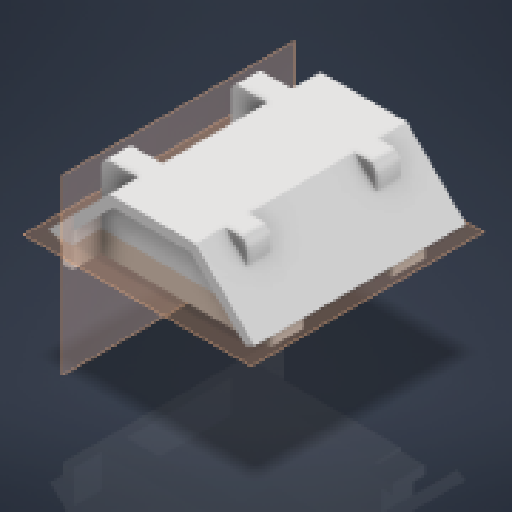
# Autodesk Inventor part: КрышкаЕСК
Saved by Autodesk Inventor 2026 (Build 300175000, 175)
## iProperties
Created: 2025-08-21
Part Number: КрышкаЕСК
Material: Типовые
Document SubType Name: Modeling
Designer: seraf
Density: 1 g/cm^3
Appearance: По умолчанию
Author: seraf
Autodesk Inventor part; units mm, degrees
ref_plane "XY Plane" through (0, 0, 0) normal (0, 0, 1) x (1, 0, 0)
sketch "Эскиз1" plane through (0, 0, 0) normal (0, 0, 1) x (1, 0, 0)
  line L0 (21.7279, 9) -> (24, 10) projected
  line L1 (10, 24) -> (24, 10) projected
  line L2 (-10, 24) -> (10, 24) projected
  line L3 (-24, 10) -> (-10, 24) projected
  line L4 (-24, 10) -> (-21.7279, 9) projected
  line L5 (-9, 21.7279) -> (-21.7279, 9) projected
  line L6 (9, 21.7279) -> (-9, 21.7279) projected
  line L7 (21.7279, 9) -> (9, 21.7279) projected
  point P0 (0, 0)
ref_plane "РабПлоскость1" through (-24, 9, 50) normal (0, 0, -1) x (0, 1, 0)
extrude "Выдавливание1" add sketch "Эскиз1" along normal up to surface (50 mm away)
sketch "Эскиз2" plane through (0, 0, 0) normal (0, 0, -1) x (-1, 0, 0)
  line L0 (-21.7279, 9) -> (-24, 10) projected
  line L1 (-10, 24) -> (-24, 10) projected
  line L2 (10, 24) -> (-10, 24) projected
  line L3 (24, 10) -> (10, 24) projected
  line L4 (24, 10) -> (21.7279, 9) projected
  line L5 (9, 21.7279) -> (21.7279, 9) projected
  line L6 (-9, 21.7279) -> (9, 21.7279) projected
  line L7 (-21.7279, 9) -> (-9, 21.7279) projected
  point P0 (0, 0)
extrude "Выдавливание2" cut sketch "Эскиз2" against normal blind 0.5
sketch "Эскиз4" plane through (-10, 24, 50) normal (0, 0, 1) x (1, 0, 0)
  line L0 (19, -2.2721) -> (31.7279, -15) projected
  line L1 (31.7279, -15) -> (34, -14) projected
  line L2 (34, -14) -> (20, 0) projected
  line L3 (20, 0) -> (0, 0) projected
  line L4 (0, 0) -> (-14, -14) projected
  line L5 (-14, -14) -> (-11.7279, -15) projected
  line L6 (-11.7279, -15) -> (1, -2.2721) projected
  line L7 (1, -2.2721) -> (19, -2.2721) projected
  point P0 (10, -24)
extrude "Выдавливание4" cut sketch "Эскиз4" against normal blind 0.5
ref_plane "РабПлоскость3" through (-18.5, 0, 0) normal (1, 0, 0) x (0, 1, 0)
sketch "Эскиз6" plane through (-18.5, 0, 0) normal (1, 0, 0) x (0, 1, 0)
  circle A0 centre (7.1085, 40) radius 1.5 projected
  circle A1 centre (7.1085, 10) radius 1.5 projected
  line L0 (-9, 55) -> (9, 55) construction
  line L1 (-9, 55) -> (-9, -15) construction
  line L2 (9, -15) -> (-9, -15) construction
  line L3 (9, 0) -> (9, -15) construction
  line L4 (9, 50) -> (9, 0) construction
  line L5 (9, 55) -> (9, 50) construction
  line L6 (9, 0.5) -> (9, 49.5) projected
  line L7 (9, 49.5) -> (4.5, 49.5)
  line L8 (4.5, 49.5) -> (4.5, 0.5)
  line L9 (4.5, 0.5) -> (9, 0.5)
  line L10 (9, 0.5) -> (9, 49.5)
  point P0 (0, 0)
  dimension "d10" = 4.5
  constraints: 8 end point, 2 parallel, 1 horizontal, 1 perpendicular
  measures "d10" distance of L9.end L8.end
extrude "Выдавливание5" add sketch "Эскиз6" against normal blind 2.5
sketch "Эскиз7" plane through (-18.5, 9, 49.5) normal (0, 1, 0) x (1, 0, 0)
  line L0 (0, 49) -> (0, 0) projected
  line L1 (0, 49) -> (-2.5, 49) projected
  line L2 (-2.5, 0) -> (-2.5, 49) projected
  line L3 (0, 0) -> (-2.5, 0) projected
  point P0 (18.5, 49.5)
extrude "Выдавливание6" add sketch "Эскиз7" along normal up to surface surface through (-21.7279, 9, 0) normal (0.7071068, -0.7071068, 0)
sketch "Эскиз8" plane through (-21.7279, 9, 49.5) normal (0.7071068, -0.7071068, 0) x (-0.7071068, -0.7071068, 0)
  line L0 (-1.0294, 49) -> (-1.0294, 0) projected
  line L1 (-1.0294, 0) -> (0, 0) projected
  line L2 (0, 49) -> (0, 0) projected
  line L3 (0, 49) -> (-1.0294, 49) projected
  point P0 (-9, 49.5)
extrude "Выдавливание7" add sketch "Эскиз8" along normal up to surface surface through (-21, 6.75, 25) normal (1, 0, 0)
sketch "Эскиз9" plane through (-21, 7.1085, 10) normal (1, 0, 0) x (0, 0, -1)
  circle A0 centre (-30, 0) radius 1.5 projected
  circle A1 centre (0, 0) radius 1.5 projected
  point P0 (10, -7.1085)
extrude "Выдавливание8" cut sketch "Эскиз9" against normal blind 10
ref_plane "РабПлоскость4" through (0, 9.5, 0) normal (0, 1, 0) x (-1, 0, 0)
sketch "Эскиз10" plane through (0, 9.5, 0) normal (0, 1, 0) x (-1, 0, 0)
  line L0 (-21.7279, 15.2) -> (-21.7279, 6.8) construction
  line L1 (-21.7279, 43.2) -> (-21.7279, 34.8) construction
  line L2 (-18.7279, 6.8) -> (-18.7279, 15.2) construction
  line L3 (-18.7279, 34.8) -> (-18.7279, 43.2) construction
  line L4 (-18.2279, 7.2) -> (-15.2279, 7.2)
  line L5 (-15.2279, 7.2) -> (-15.2279, 14.8)
  line L6 (-15.2279, 14.8) -> (-18.2279, 14.8)
  line L7 (-18.2279, 14.8) -> (-18.2279, 7.2)
  line L8 (-18.2279, 35.2) -> (-15.2279, 35.2)
  line L9 (-15.2279, 35.2) -> (-15.2279, 42.8)
  line L10 (-15.2279, 42.8) -> (-18.2279, 42.8)
  line L11 (-18.2279, 42.8) -> (-18.2279, 35.2)
  line L12 (-18.7279, 14.8) -> (-18.2279, 14.8) construction
  line L13 (-18.7279, 42.8) -> (-18.2279, 42.8) construction
  line L14 (-24, 55) -> (-24, -15) construction
  point P0 (0, 0)
  dimension "d20" = 0.5
  dimension "d21" = 3
  dimension "d26" = 7.6
  dimension "d27" = 0.4
  dimension "d28" = 0.4
  dimension "d29" = 7.6
  constraints: 20 end point, 6 parallel, 4 horizontal, 2 perpendicular, 2 point on line
  measures "d20" distance of L12.start L6.end
  measures "d21" distance of L5.end L6.end
  measures "d26" distance of L4.end L5.end
  measures "d27" distance of L2.end L12.start
  measures "d28" distance of L3.end L13.start
  measures "d29" distance of L8.end L9.end
extrude "Выдавливание9" add sketch "Эскиз10" along normal up to surface surface through (9, 21.7279, 0) normal (-0.7071068, -0.7071068, 0)
sketch "Эскиз11" plane through (0, 9.5, 0) normal (0, -1, 0) x (1, 0, 0)
  line L0 (15.2279, 7.2) -> (15.2279, 14.8) projected
  line L1 (18.2279, 7.2) -> (15.2279, 7.2) projected
  line L2 (18.2279, 14.8) -> (18.2279, 7.2) projected
  line L3 (15.2279, 14.8) -> (18.2279, 14.8) projected
  line L4 (15.2279, 35.2) -> (15.2279, 42.8) projected
  line L5 (18.2279, 35.2) -> (15.2279, 35.2) projected
  line L6 (18.2279, 42.8) -> (18.2279, 35.2) projected
  line L7 (15.2279, 42.8) -> (18.2279, 42.8) projected
  point P0 (0, 0)
extrude "Выдавливание10" add sketch "Эскиз11" along normal blind 4.25
sketch "Эскиз12" plane through (18.2279, 12.5, 14.8) normal (1, 0, 0) x (0, 0, -1)
  line L0 (-20.4, -7.25) -> (-28, -7.25) projected
  line L1 (7.6, -7.25) -> (0, -7.25) projected
  line L2 (-28, -7.25) -> (-28, 0) projected
  line L3 (-20.4, -7.25) -> (-20.4, 0) projected
  line L4 (-28, -7.25) -> (-20.4, -7.25)
  line L5 (-20.4, -7.25) -> (-20.4, -5)
  line L6 (-20.4, -5) -> (-28, -5)
  line L7 (-28, -5) -> (-28, -7.25)
  line L8 (7.6, 3) -> (7.6, -7.25) projected
  line L9 (0, -7.25) -> (7.6, -7.25)
  line L10 (7.6, -7.25) -> (7.6, -5)
  line L11 (7.6, -5) -> (0, -5)
  line L12 (0, -5) -> (0, -7.25)
  point P0 (14.8, -12.5)
  point P1 (-28, -5)
  dimension "d30" = 2.25
  dimension "d31" = 2.25
  constraints: 16 end point, 4 parallel, 2 horizontal, 2 perpendicular, 2 point on line
  measures "d30" distance of L5.end L4.end
  measures "d31" distance of L10.end L9.end
extrude "Выдавливание11" add sketch "Эскиз12" along normal blind 2.5
sketch "Эскиз13" plane through (21.7279, 9, 0.5) normal (0.402835, -0.9152726, 0) x (0.9152726, 0.402835, 0)
  line L0 (0, 0) -> (2.4824, 0) projected
  line L1 (2.4824, 0) -> (2.4824, 49) projected
  line L2 (0, 0) -> (0, 49) projected
  line L3 (2.4824, 49) -> (0, 49) projected
  point P0 (-23.5125, -0.5)
extrude "Выдавливание12" cut sketch "Эскиз13" against normal blind 0.4 draft 40
sketch "Эскиз14" plane through (-18.5, 4.5, 0.5) normal (0, -1, 0) x (1, 0, 0)
  circle A0 centre (33.25, 35) radius 1.5 construction
  circle A1 centre (33.25, 35) radius 1.5 construction
  line L0 (33.7279, 42.3) -> (33.7279, 34.7) construction
  line L1 (33.7279, 14.3) -> (33.7279, 6.7) construction
  line L2 (0, 49) -> (0, 0) construction
  line L3 (33.7279, 42.3) -> (0, 42.3)
  line L4 (0, 42.3) -> (0, 36.7)
  line L5 (0, 36.7) -> (33.7279, 36.7)
  line L6 (33.7279, 36.7) -> (33.7279, 42.3)
  line L7 (33.7279, 12.3) -> (0, 12.3)
  line L8 (0, 12.3) -> (0, 6.7)
  line L9 (0, 6.7) -> (33.7279, 6.7)
  line L10 (33.7279, 6.7) -> (33.7279, 12.3)
  point P0 (18.5, -0.5)
  dimension "d36" = 2
  dimension "d39" = 2
  constraints: 16 end point, 4 parallel, 3 point on line, 2 horizontal, 2 perpendicular
  measures "d36" distance of L1.start L7.start
  measures "d39" distance of L5.end L0.end
extrude "Выдавливание13" add sketch "Эскиз14" against normal up to surface (19.5 mm away)
sketch "Эскиз15" plane through (-18.5, 7.1085, 40) normal (-1, 0, 0) x (0, 0, 1)
  circle A0 centre (0, 0) radius 1.5 projected
  circle A1 centre (-30, 0) radius 1.5 projected
  point P0 (-40, -7.1085)
extrude "Выдавливание14" cut sketch "Эскиз15" against normal blind 5
fillet "Сопряжение1" radius 2 4 edges at (-18.5, 24, 10) (-18.5, 24, 40) (15.2279, 24, 40) (15.2279, 24, 10)
